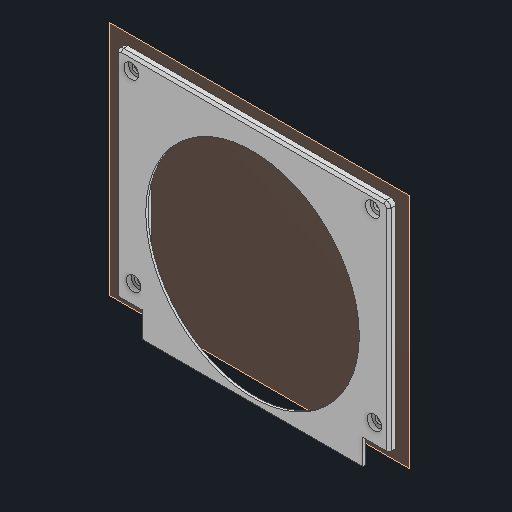
# Autodesk Inventor part: BP_FanCover
Saved by Autodesk Inventor 2026.1 (Build 301233020, 233B)
## iProperties
Created: 2025-09-13
Part Number: BP_FanCover
Material: Generic
Document SubType Name: Modeling
Designer: atrus
Density: 1 g/cm^3
Appearance: Default
Author: atrus
Autodesk Inventor part; units mm, degrees
ref_plane "YZ Plane" through (0, 0, 0) normal (1, 0, 0) x (0, 1, 0)
ref_plane "XZ Plane" through (0, 0, 0) normal (0, 1, 0) x (-1, 0, 0)
ref_plane "XY Plane" through (0, 0, 0) normal (0, 0, 1) x (1, 0, 0)
ref_plane "Work Plane1" through (0, 0, -0.1) normal (0, 0, 1) x (1, 0, 0)
sketch "Sketch1" plane through (0, 0, -0.1) normal (0, 0, 1) x (1, 0, 0)
  circle A0 centre (-100.824, -72) radius 2
  circle A1 centre (2.867, -72) radius 2
  circle A2 centre (-101.9061, 6.8071) radius 2
  circle A3 centre (2.0738, 7.307) radius 2
  spline S0 degree 3 poles (-108.332, 10.6) (-108.332, 10.8554) (-108.2821, 11.108) (-108.0875, 11.5833) (-107.9438, 11.8006) (-107.5783, 12.1734) (-107.3584, 12.3239) (-106.9863, 12.4852) (-106.8508, 12.528) (-106.5731, 12.5855) (-106.4315, 12.6) (-106.2896, 12.6) knots 0 0 0 0 0.240766 0.240766 0.484156 0.484156 0.732838 0.732838 0.866308 0.866308 1 1 1 1
  line L0 (-108.332, 10.6) -> (-108.332, -80)
  line L1 (-96.066, -80) -> (-108.332, -80)
  line L2 (-96.066, -80) -> (-96.066, 1.6)
  arc A4 (-94.066, 3.6) -> (-96.066, 1.6) centre (-94.066, 1.6) ccw
  line L3 (-94.066, 3.6) -> (-5.266, 3.6)
  arc A5 (-3.266, 1.6) -> (-5.266, 3.6) centre (-5.266, 1.6) ccw
  line L4 (-3.266, -80) -> (-3.266, 1.6)
  line L5 (-3.266, -80) -> (9, -80)
  line L6 (9, 10.6) -> (9, -80)
  spline S1 degree 3 poles (6.9576, 12.6) (7.2289, 12.6) (7.4978, 12.5471) (7.9966, 12.3419) (8.2225, 12.1926) (8.5986, 11.8187) (8.7467, 11.5995) (8.9481, 11.1175) (9, 10.8602) (9, 10.6) knots 0 0 0 0 0.255338 0.255338 0.507826 0.507826 0.754805 0.754805 1 1 1 1
  line L7 (-106.2896, 12.6) -> (6.9576, 12.6)
  point P0 (0, 0)
extrude "Extrusion1" add sketch "Sketch1" along normal blind 2 contours A0 | A1 | A2 | A3 | S0 L7 S1 L6 L5 L4 A5 L3 A4 L2 L1 L0
sketch "Sketch2" plane through (0, 0, 1.9) normal (0, 0, 1) x (1, 0, 0)
  line L0 (9, -80) -> (9, 10.6) projected
  ellipse E0 centre (6.9576, 10.6) end of major axis (9, 10.6) minor radius 2 (9, 10.6) -> (6.9576, 12.6) ccw projected
  line L1 (6.9576, 12.6) -> (-106.2896, 12.6) projected
  ellipse E1 centre (-106.2896, 10.6) end of major axis (-104.2473, 10.5998) minor radius 2 (-106.2896, 12.6) -> (-108.332, 10.6) ccw projected
  line L2 (-108.332, 10.6) -> (-108.332, -80) projected
  line L3 (8.2, -80) -> (8.2, 10.6)
  line L4 (6.9576, 11.8) -> (-106.2896, 11.8)
  line L5 (-107.532, 10.6) -> (-107.532, -80)
  circle A0 centre (-49.666, -42.9) radius 0.5 projected
  circle A1 centre (-49.666, -42.9) radius 46
  line L6 (8.2, -80) -> (-2.2, -80)
  line L7 (-2.2, -80) -> (-2.2, -90.9)
  line L8 (-2.2, -90.9) -> (-97.166, -90.9)
  line L9 (-97.166, -90.9) -> (-97.166, -80)
  line L10 (-97.166, -80) -> (-107.532, -80)
  line L11 (-97.366, -98.2561) -> (-97.366, -79.6439) construction
  line L12 (-2, -79.6439) -> (-2, -98.2561) construction
  spline S0 degree 4 poles (8.2, 10.6) (8.1999, 10.8352) (8.1361, 11.0703) (7.879, 11.4945) (7.4469, 11.738) (7.2023, 11.8) (6.9576, 11.8) knots 0 0 0 0 0 0.490114 0.490114 1 1 1 1 1
  spline S1 degree 4 poles (-106.2896, 11.8) (-106.5343, 11.8) (-106.7789, 11.738) (-107.211, 11.4945) (-107.4681, 11.0703) (-107.5319, 10.8352) (-107.532, 10.6) knots 0 0 0 0 0 0.509886 0.509886 1 1 1 1 1
  point P0 (0, 0)
  point P1 (-96.066, -80)
  point P2 (-3.266, -80)
  dimension "d2" = 0.8
  dimension "d3" = 92
  dimension "d6" = 48
  dimension "d18" = 0.2
  dimension "d24" = 0.2
  constraints: 16 end point, 5 parallel, 3 perpendicular, 2 point on line, 1 centre point, 1 coincident, 1 horizontal, 8 other
  measures "d2" distance between parallel lines of L0 L3
  measures "d3" diameter of A1
  measures "d6" distance from line of L8 A0.centre
  measures "d18" distance between parallel lines of L11 L9
  measures "d24" distance between parallel lines of L12 L7
extrude "Extrusion2" add sketch "Sketch2" along normal blind 1 contours L6 L7 L8 L9 L10 L5 S1 L4 S0 L3
sketch "Sketch3" plane through (0, 0, 2.9) normal (0, 0, 1) x (1, 0, 0)
  circle A0 centre (2.0738, 7.307) radius 2 construction
  circle A1 centre (2.867, -72) radius 2 construction
  circle A2 centre (-100.824, -72) radius 2 construction
  circle A3 centre (-101.9061, 6.8071) radius 2 construction
  point P0 (0, 0)
  constraints: 4 coincident
hole "Hole1" at (2.0738, 7.307, 2.9) at (-101.9061, 6.8071, 2.9) at (-100.824, -72, 2.9) at (2.867, -72, 2.9) direction (0, 0, -1) diameter 3.4 end through all counterbore diameter 6.3 counterbore depth 2 clearance for "Flat Head Machine Screw" size "M3" standard "Ansi Metric M Profile"
sketch "Sketch4" plane through (0, 0, 1.9) normal (0, 0, 1) x (1, 0, 0)
  line L0 (8.2, 10.6) -> (8.2, -80) projected
  line L1 (8.2, -80) -> (9, -80) projected
  line L2 (9, -80) -> (9, 10.6) projected
  ellipse E0 centre (6.9576, 10.6) end of major axis (9, 10.6) minor radius 2 (9, 10.6) -> (6.9576, 12.6) ccw projected
  line L3 (6.9576, 12.6) -> (-106.2896, 12.6) projected
  ellipse E1 centre (-106.2896, 10.6) end of major axis (-104.2473, 10.5998) minor radius 2 (-106.2896, 12.6) -> (-108.332, 10.6) ccw projected
  line L4 (-108.332, 10.6) -> (-108.332, -80) projected
  line L5 (-108.332, -80) -> (-107.532, -80) projected
  line L6 (-107.532, -80) -> (-107.532, 10.6) projected
  ellipse E2 centre (-106.2908, 10.6011) end of major axis (-105.0496, 10.6165) minor radius 1.1989 (-106.2896, 11.8) -> (-107.532, 10.6) ccw projected
  line L7 (-106.2896, 11.8) -> (6.9576, 11.8) projected
  ellipse E3 centre (6.9588, 10.6011) end of major axis (8.1999, 10.5856) minor radius 1.1989 (8.2, 10.6) -> (6.9576, 11.8) ccw projected
  point P0 (0, 0)
  constraints: 4 other
extrude "Extrusion3" add sketch "Sketch4" along normal blind 1
chamfer "Chamfer1" distance 1 angle 45 5 edges at (-49.666, 12.6, 2.9) (-107.7338, 12.0142, 2.9) (-108.332, -34.7, 2.9) (8.4018, 12.0142, 2.9) (9, -34.7, 2.9)
body "Solid1"
